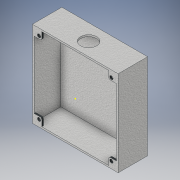
# Autodesk Inventor part: Button box back part
Saved by Autodesk Inventor 2018 (Build 220112000, 112)
## iProperties
Created: 2019-09-19
Part Number: Button box back part
Material: Aluminum 6061
Document SubType Name: Modeling
Designer: Jacob
Density: 2.7 g/cm^3
Appearance: Aluminum - Flat
Author: Jacob
Autodesk Inventor part; units mm, degrees
ref_plane "YZ Plane" through (0, 0, 0) normal (1, 0, 0) x (0, 1, 0)
ref_plane "XZ Plane" through (0, 0, 0) normal (0, 1, 0) x (-1, 0, 0)
ref_plane "XY Plane" through (0, 0, 0) normal (0, 0, 1) x (1, 0, 0)
sketch "Sketch1" plane through (0, 0, 0) normal (0, 0, 1) x (1, 0, 0)
  line L0 (-50.8, 50.8) -> (50.8, 50.8)
  line L1 (50.8, 50.8) -> (50.8, -50.8)
  line L2 (50.8, -50.8) -> (-50.8, -50.8)
  line L3 (-50.8, -50.8) -> (-50.8, 50.8)
  line L4 (-50.8, 50.8) -> (50.8, -50.8) construction
  line L5 (50.8, 50.8) -> (-50.8, -50.8) construction
  point P0 (0, 0)
  dimension "d0" = 101.6
  dimension "d1" = 101.6
  constraints: 12 end point, 2 midpoint, 2 parallel, 1 horizontal, 1 perpendicular
  measures "d0" distance of L0.start L0.end
  measures "d1" distance of L0.end L1.end
extrude "Extrusion1" add sketch "Sketch1" along normal blind 3.175
sketch "Sketch2" plane through (0, 0, 3.175) normal (0, 0, 1) x (1, 0, 0)
  line L0 (-48.768, 48.768) -> (48.768, 48.768)
  line L1 (48.768, 48.768) -> (48.768, -48.768)
  line L2 (48.768, -48.768) -> (-48.768, -48.768)
  line L3 (-48.768, -48.768) -> (-48.768, 48.768)
  line L4 (-48.768, 48.768) -> (48.768, -48.768) construction
  line L5 (48.768, 48.768) -> (-48.768, -48.768) construction
  line L6 (50.8, 50.8) -> (-50.8, 50.8) projected
  line L7 (-50.8, -50.8) -> (50.8, -50.8) projected
  line L8 (-50.8, 50.8) -> (50.8, 50.8)
  line L9 (50.8, 50.8) -> (50.8, -50.8)
  line L10 (50.8, -50.8) -> (-50.8, -50.8)
  line L11 (-50.8, -50.8) -> (-50.8, 50.8)
  point P0 (0, 0)
  dimension "d4" = 2.032
  dimension "d5" = 2.032
  constraints: 20 end point, 4 parallel, 2 horizontal, 2 midpoint, 2 perpendicular
  measures "d4" distance between parallel lines of L6 L0
  measures "d5" distance between parallel lines of L9 L1
extrude "Extrusion2" add sketch "Sketch2" along normal blind 31.75
sketch "Sketch5" plane through (-48.768, 48.768, 3.175) normal (0, -1, 0) x (1, 0, 0)
  line L0 (0, 0) -> (0, 31.75) projected
  line L1 (97.536, 0) -> (97.536, 31.75) projected
  line L2 (0, 31.75) -> (97.536, 31.75) projected
  line L3 (97.536, 0) -> (0, 0) projected
  line L4 (0, 15.875) -> (97.536, 15.875) construction
  line L5 (48.768, 15.875) -> (48.768, 31.75) construction
  line L6 (48.768, 15.875) -> (48.768, 0) construction
  circle A0 centre (48.768, 15.875) radius 9.525
  point P0 (48.768, -3.175)
  dimension "d9" = 19.05
  constraints: 6 end point, 5 midpoint, 1 centre point, 1 coincident
  measures "d9" diameter of A0
extrude "Extrusion3" cut sketch "Sketch5" against normal blind 25.4 contours A0
sketch "Sketch6" plane through (0, 0, 34.925) normal (0, 0, 1) x (1, 0, 0)
  point P0 (0, 0)
sketch "Sketch7" plane through (0, 0, 34.925) normal (0, 0, 1) x (1, 0, 0)
  line L0 (-50.8, 50.8) -> (50.8, 50.8) projected
  line L1 (0, 50.8) -> (0, -50.8) construction
  line L2 (50.8, -50.8) -> (-50.8, -50.8) projected
  line L3 (-50.8, -50.8) -> (-50.8, 50.8) projected
  line L4 (-50.8, 0) -> (50.8, 0) construction
  line L5 (50.8, -50.8) -> (50.8, 50.8) projected
  line L6 (-50.8, 42.8625) -> (50.8, 42.8625) construction
  circle A0 centre (-42.8625, 42.8625) radius 2
  circle A1 centre (42.8625, 42.8625) radius 2
  line L7 (-50.8, -42.8625) -> (50.8, -42.8625) construction
  circle A2 centre (-42.8625, -42.8625) radius 2
  circle A3 centre (42.8625, -42.8625) radius 2
  line L8 (-48.768, -48.768) -> (-48.768, 48.768) projected
  line L9 (-48.768, 48.768) -> (-39.6875, 48.768)
  line L10 (-39.6875, 48.768) -> (-39.6875, 39.6875)
  line L11 (-39.6875, 39.6875) -> (-48.768, 39.6875)
  line L12 (-48.768, 39.6875) -> (-48.768, 48.768)
  line L13 (48.768, 48.768) -> (-48.768, 48.768) projected
  line L14 (48.768, 48.768) -> (39.6875, 48.768)
  line L15 (39.6875, 48.768) -> (39.6875, 39.6875)
  line L16 (39.6875, 39.6875) -> (48.768, 39.6875)
  line L17 (48.768, 39.6875) -> (48.768, 48.768)
  line L18 (-48.768, -48.768) -> (-39.6875, -48.768)
  line L19 (-39.6875, -48.768) -> (-39.6875, -39.6875)
  line L20 (-39.6875, -39.6875) -> (-48.768, -39.6875)
  line L21 (-48.768, -39.6875) -> (-48.768, -48.768)
  line L22 (48.768, -48.768) -> (48.768, 48.768) projected
  line L23 (48.768, -48.768) -> (39.6875, -48.768)
  line L24 (39.6875, -48.768) -> (39.6875, -39.6875)
  line L25 (39.6875, -39.6875) -> (48.768, -39.6875)
  line L26 (48.768, -39.6875) -> (48.768, -48.768)
  point P0 (0, 0)
  dimension "d12" = 85.725
  dimension "d13" = 4
  dimension "d14" = 4
  dimension "d16" = 85.725
  dimension "d17" = 42.8625
  dimension "d18" = 42.8625
  dimension "d19" = 4
  dimension "d20" = 4
  dimension "d21" = 42.8625
  dimension "d22" = 42.8625
  dimension "d23" = 85.725
  dimension "d24" = 42.8625
  dimension "d25" = 42.8625
  dimension "d26" = 3.175
  dimension "d27" = 3.175
  dimension "d28" = 3.175
  dimension "d29" = 3.175
  dimension "d30" = 3.175
  dimension "d31" = 3.175
  dimension "d32" = 3.175
  dimension "d33" = 3.175
  constraints: 40 end point, 8 parallel, 8 point on line, 6 perpendicular, 4 centre point, 4 horizontal, 4 midpoint
  measures "d12" distance of A1.centre A0.centre
  measures "d13" diameter of A0
  measures "d14" diameter of A1
  measures "d16" distance of A3.centre A2.centre
  measures "d17" distance from line of L1 A0.centre
  measures "d18" distance from line of L1 A1.centre
  measures "d19" diameter of A2
  measures "d20" diameter of A3
  measures "d21" distance from line of L1 A2.centre
  measures "d22" distance from line of L1 A3.centre
  measures "d23" distance between parallel lines of L7 L6
  measures "d24" distance between parallel lines of L4 L6
  measures "d25" distance between parallel lines of L4 L7
  measures "d26" distance from line of L10 A0.centre
  measures "d27" distance from line of L11 A0.centre
  measures "d28" distance from line of L15 A1.centre
  measures "d29" distance from line of L16 A1.centre
  measures "d30" distance from line of A2.centre L20
  measures "d31" distance from line of L19 A2.centre
  measures "d32" distance from line of L25 A3.centre
  measures "d33" distance from line of L24 A3.centre
extrude "Extrusion4" add sketch "Sketch7" against normal blind 2 contours L8 L20 L19 L18 | L8 L9 L10 L11 | L17 L16 L15 L13 | L23 L24 L25 L22
fillet "Fillet1" radius 2 4 edges at (-39.6875, 39.6875, 33.925) (39.6875, 39.6875, 33.925) (39.6875, -39.6875, 33.925) (-39.6875, -39.6875, 33.925)
equation "\"d17\" = d18"
equation "\"d21\" = d22"
equation "\"d24\" = d25"
body "Solid1"
